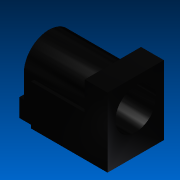
# Autodesk Inventor part: 2.1mm DC Power Socket Housing
Saved by Autodesk Inventor 2013 (Build 170138000, 138)
## iProperties
Created: 2012-05-07
Material: ABS Plastic
Document SubType Name: Modeling
Designer: sdarley
Density: 1 g/cm^3
Project: 2.1mm DC Power Socket
Description: 2.1mm DC Power Socket Housing
Author: sdarley
Title: 2.1mm DC Power Socket Housing
Revision Number: 1
Autodesk Inventor part; units mm, degrees
ref_plane "YZ Plane" through (0, 0, 0) normal (1, 0, 0) x (0, 1, 0)
ref_plane "XZ Plane" through (0, 0, 0) normal (0, 1, 0) x (-1, 0, 0)
ref_plane "XY Plane" through (0, 0, 0) normal (0, 0, 1) x (1, 0, 0)
sketch "Sketch1" plane through (0, 0, 0) normal (1, 0, 0) x (0, 1, 0)
  line L0 (-4.375, 0) -> (4.375, 0)
  line L1 (4.375, 0) -> (4.375, 10.75)
  line L2 (4.375, 10.75) -> (-4.375, 10.75)
  line L3 (-4.375, 10.75) -> (-4.375, 0)
  circle A0 centre (0, 6.4) radius 3.15
  point P0 (0, 0)
  point P1 (0, 10.75)
  dimension "d0" = 8.75
  dimension "d1" = 10.75
  dimension "d2" = 6.3
  dimension "d3" = 1.2
  constraints: 8 end point, 2 parallel, 2 vertical alignment, 1 centre point, 1 horizontal, 1 midpoint, 1 perpendicular
  measures "d0" distance of L2.end L1.end
  measures "d1" distance of L1.end L0.end
  measures "d2" diameter of A0
  measures "d3" distance edge to line of A0 L2
extrude "Extrusion1" add sketch "Sketch1" along normal blind 3.55
sketch "Sketch2" plane through (0, 0, 0) normal (-1, 0, 0) x (0, 0, 1)
  circle A0 centre (6.4, 0) radius 3.15 projected
  line L0 (0, -4.375) -> (0, 4.375) projected
  line L1 (10.75, -4.375) -> (0, -4.375) projected
  line L2 (0, 4.375) -> (10.75, 4.375) projected
  line L3 (6.3, 4.375) -> (6.3, 3.1484)
  line L4 (6.3, -3.1484) -> (6.3, -4.375)
  point P0 (0, 0)
  dimension "d7" = 6.3
  constraints: 4 end point, 2 perpendicular, 2 point on circle, 2 point on line, 1 vertical alignment
  measures "d7" distance between parallel lines of L3 L0
extrude "Extrusion2" add sketch "Sketch2" along normal blind 8.35 contours A0 L4 L1 L0 L2 L3
sketch "Sketch3" plane through (-8.35, 0, 0) normal (-1, 0, 0) x (0, 0, 1)
  line L0 (6.3, -4.375) -> (6.3, -3.1484) projected
  arc A0 (6.3, 3.1484) -> (6.3, -3.1484) centre (6.4, 0) ccw projected
  line L1 (6.3, 3.1484) -> (6.3, 4.375) projected
  arc A1 (6.3, -3.8737) -> (6.3, 3.8737) centre (6.4, 0) ccw
  arc A2 (6.3, -3.1484) -> (6.3, 3.1484) centre (6.4, 0) ccw projected
  line L2 (6.3, 3.8737) -> (6.3, 3.1484)
  line L3 (6.3, -3.1484) -> (6.3, -3.8737)
  point P0 (0, 0)
  dimension "d10" = 3.875
  constraints: 4 end point, 3 point on circle, 1 centre point, 1 coincident, 1 collinear, 1 point on line
  measures "d10" radius of A1
extrude "Extrusion3" add sketch "Sketch3" against normal up to next contours L0 A2 L1 A1
sketch "Sketch4" plane through (-8.35, 0, 0) normal (-1, 0, 0) x (0, 0, 1)
  circle A0 centre (6.4, 0) radius 3.15 projected
  point P0 (0, 0)
extrude "Extrusion4" add sketch "Sketch4" against normal blind 2.55
sketch "Sketch5" plane through (-8.35, 0, 0) normal (-1, 0, 0) x (0, 0, 1)
  line L0 (6.3, 4.375) -> (0, 4.375) projected
  line L1 (0, 4.375) -> (0, -4.375) projected
  line L2 (6.3, -4.375) -> (6.3, -3.8737) projected
  arc A0 (6.3, -3.8737) -> (6.3, 3.8737) centre (6.4, 0) ccw projected
  line L3 (7.05, 3.8201) -> (7.05, 2.225)
  line L4 (7.05, 2.225) -> (4.9, 2.225)
  line L5 (4.9, 2.225) -> (4.9, 3.675)
  line L6 (4.9, 3.675) -> (0, 3.675)
  line L7 (6.3, -3.8737) -> (0, -3.8737)
  line L8 (0, 3.675) -> (0, -3.8737)
  arc A1 (6.3, -3.8737) -> (7.05, 3.8201) centre (6.4, 0) ccw
  point P0 (0, 0)
  dimension "d15" = 2.15
  dimension "d17" = 4.9
  dimension "d18" = 0.7
  dimension "d19" = 2.15
  constraints: 12 end point, 3 perpendicular, 3 point on circle, 2 parallel, 2 point on line, 1 centre point, 1 coincident, 1 collinear
  measures "d15" distance between parallel lines of L5 L3
  measures "d17" distance between parallel lines of L1 L5
  measures "d18" distance between parallel lines of L0 L6
  measures "d19" distance between parallel lines of L0 L4
extrude "Extrusion5" add sketch "Sketch5" along normal blind 1.6
sketch "Sketch6" plane through (-9.95, 0, 0) normal (-1, 0, 0) x (0, 0, 1)
  line L0 (0, 3.675) -> (0, -3.8737) projected
  line L1 (0, 3.675) -> (2.8, 3.675)
  line L2 (2.8, 3.675) -> (2.8, 1.4)
  line L3 (2.8, 1.4) -> (0, 1.4)
  line L4 (0, 1.4) -> (0, 3.675)
  line L5 (0, -3.8737) -> (2.8, -3.8737)
  line L6 (2.8, -3.8737) -> (2.8, -1.4)
  line L7 (2.8, -1.4) -> (0, -1.4)
  line L8 (0, -1.4) -> (0, -3.8737)
  arc A0 (6.3, -3.8737) -> (7.05, 3.8201) centre (6.4, 0) ccw projected
  point P0 (0, 0)
  dimension "d25" = 2.8
  dimension "d28" = 1.4
  dimension "d29" = 1.4
  constraints: 16 end point, 4 parallel, 2 horizontal, 2 perpendicular, 1 vertical alignment
  measures "d25" distance between parallel lines of L0 L2
  measures "d28" distance from line of A0.centre L3
  measures "d29" distance from line of A0.centre L7
extrude "Extrusion6" add sketch "Sketch6" along normal blind 0.7
equation "\"d29\" = d28"
body "Solid1"
